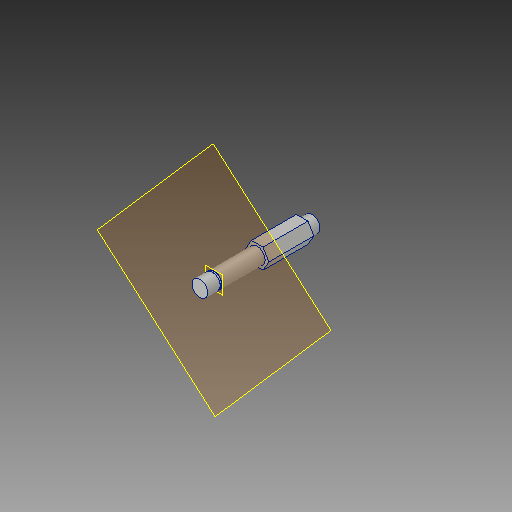
# Autodesk Inventor part: Smol Hex Shaft
Saved by Autodesk Inventor 2019.4 (Build 234330000, 330)
## iProperties
Created: 2020-01-24
Part Number: Smol Hex Shaft
Material: Aluminum 6061
Document SubType Name: Modeling
Designer: Mark
Mass: 19.7426 g
Surface Area: 28.793 cm^2
Volume: 7.31208 cm^3
Density: 2.7 g/cm^3
Appearance: Aluminum - Flat
Author: Mark
Autodesk Inventor part; units mm, degrees
ref_plane "YZ Plane" through (0, 0, 0) normal (1, 0, 0) x (0, 1, 0)
ref_plane "XZ Plane" through (0, 0, 0) normal (0, 1, 0) x (-1, 0, 0)
ref_plane "XY Plane" through (0, 0, 0) normal (0, 0, 1) x (1, 0, 0)
sketch "Sketch1" plane through (0, 0, 0) normal (0, 0, 1) x (1, 0, 0)
  line L0 (3.6662, 6.35) -> (7.3323, 0)
  line L1 (7.3323, 0) -> (3.6662, -6.35)
  line L2 (3.6662, -6.35) -> (-3.6662, -6.35)
  line L3 (-3.6662, -6.35) -> (-7.3323, 0)
  line L4 (-7.3323, 0) -> (-3.6662, 6.35)
  line L5 (-3.6662, 6.35) -> (3.6662, 6.35)
  line L6 (0, 0) -> (0, 6.35)
  line L7 (0, 0) -> (6.35, 0) construction
  dimension "d0" = 12.7
  dimension "d1" = 90
  dimension "d2" = 90
  constraints: 16 end point, 1 coincident, 1 horizontal, 1 midpoint, 1 perpendicular, 13 other
  measures "d0" distance between parallel lines of L2 L5
  measures "d1" angle of L7 L6
  measures "d2" angle of L5 L6
extrude "Extrusion1" add sketch "Sketch1" along normal blind 28.5
sketch "Sketch2" plane through (0, 0, 28.5) normal (0, 0, 1) x (1, 0, 0)
  circle A0 centre (0, 0) radius 5
  dimension "d5" = 10
  constraints: 1 centre point, 1 coincident
  measures "d5" diameter of A0
extrude "Extrusion2" add sketch "Sketch2" along normal blind 36.25
sketch "Sketch3" plane through (0, 0, 0) normal (0, 0, -1) x (-1, 0, 0)
  circle A0 centre (0, 0) radius 5
  dimension "d8" = 10
  constraints: 1 centre point, 1 coincident
  measures "d8" diameter of A0
extrude "Extrusion3" add sketch "Sketch3" along normal blind 6.25
ref_plane "Work Plane1" through (0, 0, 55.75) normal (0, 0, 1) x (1, 0, 0)
ref_plane "Work Plane2" through (0, 0, 55.75) normal (0, 0, 1) x (0.6578344, 0.7531626, 0)
sketch "Sketch4" plane through (0, 0, 55.75) normal (0, 0, 1) x (0.6578344, 0.7531626, 0)
  circle A0 centre (0, 0) radius 4.8
  circle A1 centre (0, 0) radius 5
  dimension "d12" = 9.6
  dimension "d13" = 10
  constraints: 2 centre point, 2 coincident
  measures "d12" diameter of A0
  measures "d13" diameter of A1
extrude "Extrusion4" cut sketch "Sketch4" along normal blind 1.1
body "Solid1"
